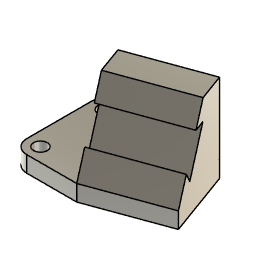
16 (Autodesk Fusion 360 design; units mm, degrees)
Autodesk Fusion 360 part; units mm, degrees
sketch "草图1" plane through (0, 0, 0) normal (1, 0, 0) x (0, 1, 0)
  line L0 (0, 0) -> (0, 1.1769)
  line L1 (0, 1.1769) -> (0, 31.1769)
  line L2 (0, 31.1769) -> (12, 31.1769)
  line L3 (12, 31.1769) -> (17.1962, 22.1769)
  line L4 (17.1962, 22.1769) -> (12.1962, 22.1769)
  line L5 (12.1962, 22.1769) -> (21.6962, 5.7224)
  line L6 (21.6962, 5.7224) -> (24.1962, 10.0526)
  line L7 (24.1962, 10.0526) -> (30, 0)
  line L8 (30, 0) -> (0, 0)
  dimension "d1" = 12
  dimension "d2" = 5
  dimension "d3" = 9
  dimension "d4" = 19
  dimension "d5" = 60
  dimension "d6" = 30
  dimension "d7" = 30
  constraint vertical L0
  constraint parallel L0 L1
  constraint perpendicular L1 L2
  constraint parallel L2 L4
  constraint parallel L3 L5
  constraint perpendicular L0 L8
  constraint coincident L0.start L8.end
  constraint parallel L3 L7
  constraint equal L4 L6
  constraint collinear L3 L7
  measures "d1" distance of L1.end L2.end
  measures "d2" distance of L3.end L4.end
  measures "d3" vertical distance of L2.end L3.end
  measures "d4" distance of L4.end L5.end
  measures "d5" angle of L4 L6
  measures "d6" distance of L0.start L7.end
  measures "d7" distance of L0.end L1.end
extrude "拉伸1" add sketch "草图1" along normal blind 4 makes body 1
move_body "移动1" bodies 1 to x (-0.939693, -0.34202, 0) y (0.34202, -0.939693, 0) z (0, 0, 1) at (1.8273, 12.3222, 0)
sketch "草图3" plane through (0, 0, 0) normal (0, 0, 1) x (1, 0, 0)
  circle A0 centre (-22, 14) radius 3
  circle A1 centre (-22, -14) radius 3
  line L0 (-28, 14) -> (-28, -14)
  line L1 (-22, 20) -> (22, 20)
  line L2 (22, 20) -> (32.2606, -8.1908)
  line L3 (32.2606, -8.1908) -> (-0.185, -20)
  line L4 (-0.185, -20) -> (-22, -20)
  line L5 (0, 24) -> (0, -24) construction
  line L6 (-25, 0) -> (29, 0) construction
  arc A2 (-28, -14) -> (-22, -20) centre (-22, -14) ccw
  arc A3 (-22, 20) -> (-28, 14) centre (-22, 14) ccw
  dimension "d10" = 12
  dimension "d11" = 6
  dimension "d12" = 44
  dimension "d13" = 28
  dimension "d14" = 110
  dimension "d15" = 30
  dimension "d16" = 22
  constraint concentric A0 A3
  constraint concentric A1 A2
  constraint horizontal L1
  constraint perpendicular L2 L3
  constraint tangent L4 A2
  constraint vertical L5
  constraint perpendicular L5 L6
  constraint symmetric A0.centre A1.centre L6
  constraint equal A2 A3
  constraint equal A0 A1
  constraint tangent L0 A3
  constraint tangent L0 A2
  constraint parallel L4 L6
  constraint tangent L1 A3
  measures "d10" diameter of A3
  measures "d11" diameter of A0
  measures "d12" distance of L1.start L1.end
  measures "d13" distance of A1.centre A0.centre
  measures "d14" angle of L1 L2
  measures "d15" distance of L1.end L2.end
  measures "d16" distance of A0.centre L5
extrude "拉伸2" add sketch "草图3" against normal blind 7 separate body makes body 2
move_body "移动2" bodies 1 to x (1, 0, 0) y (0, 1, 0) z (0, 0, 1) at (-8.5141, -2.7633, 0)
extrude "拉伸3" add 1 faces at (-2.8228, -1.0573, 9.6921) along direction (0.939693, 0.34202, 0) up to surface (30.5279 mm away) on bodies 1 bodies 1 2
sketch "草图2" plane through (0, 0, 0) normal (1, 0, 0) x (0, 1, 0)
equation "d12 = 50 mm - 6 mm"
